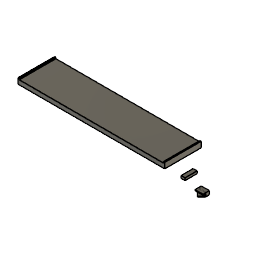
Stls iniciales (Autodesk Fusion 360 design; units mm, degrees)
Autodesk Fusion 360 part; units mm, degrees
sketch "Boceto1" plane through (0, 0, 0) normal (0, 0, 1) x (1, 0, 0)
  line L0 (0, 0) -> (50, 0)
  line L1 (50, 0) -> (50, 149.9932)
  line L2 (50, 149.9932) -> (0, 149.9932)
  line L3 (0, 149.9932) -> (0, 0)
  dimension "d1" = 50
  constraint horizontal L0
  constraint vertical L1
  constraint horizontal L2
  constraint vertical L3
  constraint coincident L0.start L3.end
  measures "d1" distance of L0.start L0.end
extrude "Extruir1" add sketch "Boceto1" along normal blind 30 makes body 1
sketch "Boceto2" plane through (0, 0, 0) normal (0, 0, 1) x (1, 0, 0)
  line L0 (-200, 0) -> (-200, 450)
  line L1 (-200, 450) -> (-2000, 450)
  line L2 (-2000, 450) -> (-2000, 0)
  line L3 (-2000, 0) -> (-200, 0)
  dimension "d6" = 450
  dimension "d7" = 1800
  constraint vertical L0
  constraint perpendicular L0 L1
  constraint perpendicular L1 L2
  constraint perpendicular L0 L3
  measures "d6" distance of L0.start L0.end
  measures "d7" distance of L0.end L1.end
extrude "Extruir2" add sketch "Boceto2" along normal blind 55 separate body makes body 2
sketch "Boceto3" plane through (0, 0, 0) normal (0, 0, 1) x (1, 0, 0)
  line L0 (250, 0) -> (350, 0)
  line L1 (350, 0) -> (350, -50)
  line L2 (250, -50) -> (250, 0)
  line L3 (350, 0) -> (250, 0)
  line L4 (250, 0) -> (250, -50)
  line L5 (250, -50) -> (350, -50)
  line L6 (350, -50) -> (350, 0)
  line L7 (350, -50) -> (300, -100)
  line L8 (300, -100) -> (250, -50)
  dimension "d10" = 100
  dimension "d12" = 50
  constraint horizontal L0
  constraint vertical L1
  constraint vertical L2
  constraint horizontal L3
  constraint vertical L4
  constraint horizontal L5
  constraint vertical L6
  constraint collinear L2 L4
  measures "d10" distance of L0.start L0.end
  measures "d12" distance of L0.end L1.end
extrude "Extruir3" add sketch "Boceto3" along normal blind 10 separate body makes body 3
sketch "Boceto4" plane through (0, 0, 10) normal (0, 0, 1) x (-1, 0, 0)
  line L0 (-350, 50) -> (-350, 0)
  line L1 (-350, 0) -> (-250, 0)
  line L2 (-250, 0) -> (-250, 50)
  line L3 (-250, 50) -> (-300, 100)
  line L4 (-300, 100) -> (-350, 50)
  line L5 (-250, 0) -> (-260, 0)
  line L6 (-260, 0) -> (-260, 45)
  line L7 (-260, 45) -> (-250, 45)
  line L8 (-250, 45) -> (-250, 0)
  line L9 (-350, 0) -> (-340, 0)
  line L10 (-340, 0) -> (-340, 45)
  line L11 (-340, 45) -> (-350, 45)
  line L12 (-350, 45) -> (-350, 0)
  line L13 (-337.5, 50) -> (-225, 50) construction
  line L14 (-260, 45) -> (-340, 45)
  line L15 (-260, 35) -> (-340, 35)
  line L16 (-262.5, 40) -> (-250, 40) construction
  line L17 (-337.5, 40) -> (-350, 40) construction
  arc A0 (-260, 30.3175) -> (-271.1603, 35) centre (-262.5, 40) ccw
  arc A1 (-328.8397, 35) -> (-340, 30.3175) centre (-337.5, 40) ccw
  dimension "d15" = 5
  dimension "d16" = 20
  dimension "d17" = 75
  dimension "d18" = 50
  dimension "d19" = 35
  dimension "d20" = 10
  constraint horizontal L5
  constraint vertical L6
  constraint horizontal L7
  constraint vertical L8
  constraint coincident L1.end L2.start
  constraint horizontal L9
  constraint vertical L10
  constraint horizontal L11
  constraint vertical L12
  constraint coincident L0.end L1.start
  constraint collinear L7 L11
  constraint equal L5 L9
  constraint equal A0 A1
  constraint coincident L13.start A1
  constraint tangent L13 A1
  constraint horizontal L13
  constraint tangent L13 A0
  constraint coincident L6 L15.start
  constraint coincident L10 L15.end
  constraint perpendicular L10 L15
  constraint coincident L16.start A0.centre
  constraint coincident L8 L16.end
  constraint coincident L17.start A1.centre
  constraint coincident L12 L17.end
  constraint equal L16 L17
  constraint horizontal L17
  constraint coincident L15 A0.end
  constraint coincident L6 A0.start
  constraint coincident L10 A1.end
  constraint coincident L15 A1.start
  measures "d15" distance of L2.end L7
  measures "d16" diameter of A0
  measures "d17" distance of L16.start L17.start
  measures "d18" distance of L1.end L13
  measures "d19" distance of L1 L15
  measures "d20" distance of L1.end L5.end
extrude "Extruir4" add sketch "Boceto4" along normal blind 25 contours L0 L1 L9 L10 L11 L12 A1 | L11 L14 A1 | L10 L11 A1 | L10 L14 L15 A1 | L14 L15 A0 A1 | L1 L2 L5 L6 L7 L8 A0 | L7 L14 A0 | L6 L14 L15 A0 | L6 L7 A0 bodies 3
sketch "Boceto5" plane through (0, 0, 35) normal (0, 0, 1) x (-1, 0, 0)
  arc A0 (-253.8397, 45) -> (-271.1603, 45) centre (-262.5, 40) ccw
  line L0 (-271.1603, 45) -> (-328.8397, 45)
  arc A1 (-328.8397, 45) -> (-346.1603, 45) centre (-337.5, 40) ccw
  line L1 (-346.1603, 45) -> (-350, 45)
  line L2 (-350, 45) -> (-350, 0)
  line L3 (-350, 0) -> (-340, 0)
  line L4 (-340, 0) -> (-340, 35)
  line L5 (-340, 35) -> (-260, 35)
  line L6 (-260, 35) -> (-260, 0)
  line L7 (-260, 0) -> (-250, 0)
  line L8 (-250, 0) -> (-250, 45)
  line L9 (-250, 45) -> (-253.8397, 45)
  line L10 (-250, 0) -> (-350, 0)
  line L11 (-350, 0) -> (-350, 80)
  line L12 (-350, 80) -> (-250, 80)
  line L13 (-250, 80) -> (-250, 0)
  dimension "d23" = 80
  constraint horizontal L10
  constraint vertical L11
  constraint horizontal L12
  constraint vertical L13
  constraint coincident L7.end L8.start
  constraint collinear L2 L11
  measures "d23" distance of L7.end L12.end
extrude "Extruir5" add sketch "Boceto5" along normal blind 10 bodies 3
sketch "Boceto6" plane through (0, 0, 55) normal (0, 0, 1) x (-1, 0, 0)
  line L0 (2000, 0) -> (200, 0)
  line L1 (200, 0) -> (200, -450)
  line L2 (200, -450) -> (2000, -450)
  line L3 (2000, -450) -> (2000, 0)
  line L4 (2000, -450) -> (1985, -450)
  line L5 (1985, -450) -> (1985, 0)
  line L6 (1985, 0) -> (2000, 0)
  line L7 (2000, 0) -> (2000, -450)
  line L8 (200, -450) -> (215, -450)
  line L9 (215, -450) -> (215, 0)
  line L10 (215, 0) -> (200, 0)
  line L11 (200, 0) -> (200, -450)
  dimension "d26" = 15
  dimension "d27" = 15
  constraint horizontal L4
  constraint vertical L5
  constraint horizontal L6
  constraint vertical L7
  constraint coincident L0 L5.end
  constraint coincident L2.end L3.start
  constraint horizontal L8
  constraint vertical L9
  constraint horizontal L10
  constraint vertical L11
  constraint coincident L0 L9.end
  constraint coincident L1.end L2.start
  measures "d26" distance of L2.end L4.end
  measures "d27" distance of L1.end L8.end
extrude "Extruir6" add sketch "Boceto6" along normal blind 15 contours L0 L2 L3 L4 L5 L6 L7 | L0 L1 L2 L8 L9 L10 L11 bodies 2
equation "d28 = 70 mm - 55 mm"
